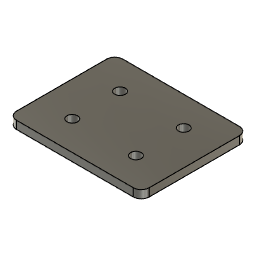
Gimballed Platform Assembly (Autodesk Fusion 360 archive; units mm, degrees)
design "Platform: gimbal"
Autodesk Fusion 360 part; units mm, degrees
sketch "Sketch1" plane through (0, 0, 0) normal (0, 0, 1) x (1, 0, 0)
  line L0 (0, 0) -> (-25, 0) construction
  line L1 (-25, 0) -> (-25, 17)
  line L2 (-22, 20) -> (0, 20)
  line L3 (0, 20) -> (0, 0) construction
  circle A0 centre (-12, 9) radius 2
  arc A1 (-22, 20) -> (-25, 17) centre (-22, 17) ccw
  circle A2 centre (-12, -9) radius 2
  arc A3 (-25, -17) -> (-22, -20) centre (-22, -17) ccw
  line L4 (-22, -20) -> (0, -20)
  line L5 (-25, 0) -> (-25, -17)
  arc A4 (25, 17) -> (22, 20) centre (22, 17) ccw
  arc A5 (22, -20) -> (25, -17) centre (22, -17) ccw
  line L6 (22, -20) -> (0, -20)
  line L7 (22, 20) -> (0, 20)
  line L8 (25, 0) -> (25, 17)
  circle A6 centre (12, -9) radius 2
  circle A7 centre (12, 9) radius 2
  line L9 (25, 0) -> (25, -17)
  point P0 (-25, 20)
  point P1 (-25, -20)
  point P2 (25, 20)
  point P3 (25, -20)
  dimension "d1" = 20
  dimension "d2" = 25
  dimension "d3" = 12
  dimension "d4" = 9
  dimension "d5" = 4
  dimension "d6" = 3
  constraint horizontal L0
  constraint vertical L1
  constraint horizontal L2
  constraint vertical L3
  constraint coincident L0.start L3.end
  constraint coincident P0 L1
  constraint coincident P0 L2
  constraint tangent L1 A1
  constraint tangent L2 A1
  constraint symmetric L3.end L0 origin
  constraint symmetric L1.start L0 L5.start
  constraint symmetric P0 L0 P1
  constraint symmetric L2.end L0 L4.end
  constraint symmetric L0 A0 A2
  constraint symmetric L0 L1.end A3.start
  constraint symmetric L0 L2.start A3.end
  constraint symmetric L0 A1 A3
  constraint symmetric L0.start L3 origin
  constraint symmetric L0.end L3 L8.start
  constraint symmetric P0 L3 P2
  constraint symmetric L2.end L3 L7.end
  constraint symmetric L3 A0 A7
  constraint symmetric L3 L1.end A4.start
  constraint symmetric L3 L2.start A4.end
  constraint symmetric L3 A1 A4
  constraint symmetric L3 L4.end L6.end
  constraint symmetric L3 L0.end L8.start
  constraint symmetric L3 L0.start origin
  constraint symmetric L3 A3.start A5.end
  constraint symmetric L3 A3.end A5.start
  constraint symmetric L3 P1 P3
  constraint symmetric L3 A2 A6
  constraint symmetric L3 A3 A5
  measures "d1" distance of L0.end P0
  measures "d2" distance of P0 L2.end
  measures "d3" distance of L3 A0.centre
  measures "d4" distance of L0 A0.centre
  measures "d5" diameter of A0
  measures "d6" radius of A1
extrude "Extrude1" add sketch "Sketch1" along normal blind 3

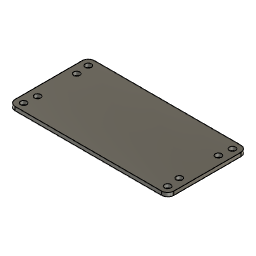
design "Platform: top"
Autodesk Fusion 360 part; units mm, degrees
sketch "Sketch1" plane through (0, 0, 0) normal (0, 0, 1) x (1, 0, 0)
  line L0 (-65, -27.5) -> (-65, 27.5)
  arc A0 (-60, 32.5) -> (-65, 27.5) centre (-60, 27.5) ccw
  arc A1 (-65, -27.5) -> (-60, -32.5) centre (-60, -27.5) ccw
  circle A2 centre (-59, 26.5) radius 2.5
  circle A3 centre (-59, -26.5) radius 2.5
  line L1 (0, 32.5) -> (0, -32.5) construction
  line L2 (-60, 32.5) -> (0, 32.5)
  line L3 (-60, -32.5) -> (0, -32.5)
  circle A4 centre (-58, 16) radius 2.5
  circle A5 centre (-58, -16) radius 2.5
  circle A6 centre (58, -16) radius 2.5
  arc A7 (60, -32.5) -> (65, -27.5) centre (60, -27.5) ccw
  line L4 (60, 32.5) -> (0, 32.5)
  circle A8 centre (59, 26.5) radius 2.5
  circle A9 centre (59, -26.5) radius 2.5
  line L5 (65, -27.5) -> (65, 27.5)
  arc A10 (65, 27.5) -> (60, 32.5) centre (60, 27.5) ccw
  circle A11 centre (58, 16) radius 2.5
  line L6 (60, -32.5) -> (0, -32.5)
  dimension "d1" = 65
  dimension "d5" = 5
  dimension "d6" = 5
  dimension "d9" = 5
  dimension "d11" = 6
  dimension "d12" = 5
  dimension "d14" = 6
  dimension "d21" = 7
  dimension "d22" = 7
  dimension "d23" = 32
  dimension "d24" = 16.5
  dimension "d25" = 65
  dimension "d28" = 5
  dimension "d29" = 5
  constraint vertical L0
  constraint tangent L0 A0
  constraint tangent L0 A1
  constraint tangent A0 L2
  constraint tangent A1 L3
  constraint symmetric A0.start L1 L4.start
  constraint symmetric L0.end L1 L5.end
  constraint symmetric A0 L1 A10
  constraint symmetric A1.end L1 A7.start
  constraint symmetric L0.start L1 A7.end
  constraint symmetric A1 L1 A7
  constraint symmetric A2 L1 A8
  constraint symmetric A3 L1 A9
  constraint symmetric L2.end L1 L4.end
  constraint symmetric L3.end L1 L6.end
  constraint symmetric L1 A4 A11
  constraint symmetric L1 A5 A6
  measures "d1" distance of origin L0
  measures "d5" radius of A0
  measures "d6" radius of A1
  measures "d9" diameter of A2
  measures "d11" distance of L0 A2.centre
  measures "d12" diameter of A3
  measures "d14" distance of L0 A3.centre
  measures "d21" distance of L0 A4.centre
  measures "d22" distance of L0 A5.centre
  measures "d23" distance of A4.centre A5.centre
  measures "d24" distance of L2 A4.centre
  measures "d25" distance of L2 L3
  measures "d28" diameter of A4
  measures "d29" diameter of A5
extrude "Extrude1" add sketch "Sketch1" along normal blind 3
equation "d6 = d5"
equation "d12 = d9"
equation "d14 = d11"
equation "d22 = d21"
equation "d24 = ( d25 - d23 ) / 2"
equation "d29 = d28"

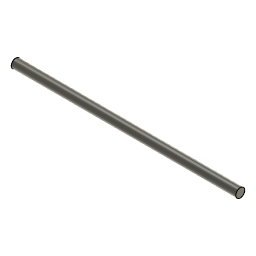
design "8mm rod"
Autodesk Fusion 360 part; units mm, degrees
sketch "Sketch1" plane through (0, 0, 0) normal (1, 0, 0) x (0, 1, 0)
  circle A0 centre (0, 0) radius 4
  dimension "d1" = 8
  constraint coincident A0.centre origin
  measures "d1" diameter of A0
extrude "Extrude1" add sketch "Sketch1" along normal blind 200
